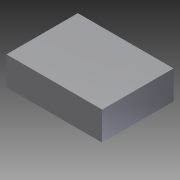
# Autodesk Inventor part: Slide switch
Saved by Autodesk Inventor 2012 (Build 160160000, 160)
## iProperties
Created: 2017-04-26
Part Number: Slide switch
Material: Default
Document SubType Name: Modeling
Designer: Brandon
Density: 1 g/cm^3
Author: Brandon
Autodesk Inventor part; units mm, degrees
ref_plane "YZ Plane" through (0, 0, 0) normal (1, 0, 0) x (0, 1, 0)
ref_plane "XZ Plane" through (0, 0, 0) normal (0, 1, 0) x (-1, 0, 0)
ref_plane "XY Plane" through (0, 0, 0) normal (0, 0, 1) x (1, 0, 0)
sketch "Sketch1" plane through (0, 0, 0) normal (0, 0, 1) x (1, 0, 0)
  line L0 (-3.35, 2) -> (3.35, 2)
  line L1 (3.35, 2) -> (3.35, 0)
  line L2 (3.35, 0) -> (-3.35, 0)
  line L3 (-3.35, 0) -> (-3.35, 2)
  point P0 (0, 0)
  dimension "d0" = 6.7
  dimension "d1" = 2
  dimension "d2" = 3.35
  dimension "d3" = 0
  constraints: 8 end point, 2 parallel, 1 horizontal, 1 perpendicular
  measures "d0" distance of L1.end L2.end
  measures "d1" distance of L0.end L1.end
  measures "d2" distance from line of point (0, 0) L3
  measures "d3" distance from line of point (0, 0) L2
extrude "Extrusion1" add sketch "Sketch1" along normal blind 5
sketch "Sketch3" plane through (-3.35, 0, 0) normal (0, -1, 0) x (1, 0, 0)
  line L0 (6.7, 5) -> (0, 5) projected
  circle A0 centre (1.85, 2.5) radius 0.4
  circle A1 centre (4.85, 2.5) radius 0.4
  point P0 (3.35, 0)
  dimension "d6" = 0.8
  dimension "d7" = 0.8
  dimension "d8" = 2.5
  dimension "d9" = 2.5
  dimension "d10" = 3
  dimension "d11" = 1.5
  constraints: 2 centre point
  measures "d6" diameter of A0
  measures "d7" diameter of A1
  measures "d8" distance from line of L0 A0.centre
  measures "d9" distance from line of L0 A1.centre
  measures "d10" distance of A1.centre A0.centre
  measures "d11" horizontal distance of point (3.35, 0) A0.centre
extrude "Extrusion2" add sketch "Sketch3" along normal blind 1.4732
equation "\"d2\" = 0.5 * d0"
body "Solid1"
